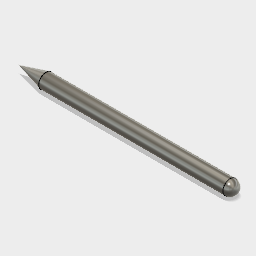
肥皂盒v1 (Autodesk Fusion 360 design; units mm, degrees)
Autodesk Fusion 360 part; units mm, degrees
cylinder "圆柱体基本要素1" add diameter 8 height 100 placed x (0, 0, -1) y (0, 1, 0) z (1, 0, 0) at (0, 53.4948, 46.5367) makes body 1
sphere "球体基本要素1" add diameter 8 placed x (1, 0, 0) y (0, 0, -1) z (0, 1, 0) at (43.301, 0, 58.6939) separate body makes body 2
move_body "对齐1" bodies 2 to x (0, 0, 1) y (0, 1, 0) z (-1, 0, 0) at (158.6939, 53.4948, 3.2357)
sketch "草图3" plane through (0, 0, 0) normal (0, 1, 0) x (1, 0, 0)
  line L0 (0, 0) -> (0, -15)
  line L1 (0, -15) -> (0, 0)
  line L2 (4, 0) -> (0, -15)
  line L3 (0, 0) -> (4, 0)
revolve "旋转1" add sketch "草图3" angle 360 about axis through (0, 0, 15) along (0, 0, -1) separate body makes body 3
move_body "对齐2" bodies 3 to x (0, 0, 1) y (0, 1, 0) z (-1, 0, 0) at (0, 53.4948, 46.5367)
combine "合并1" operation add target body 3 tool bodies 1 2
